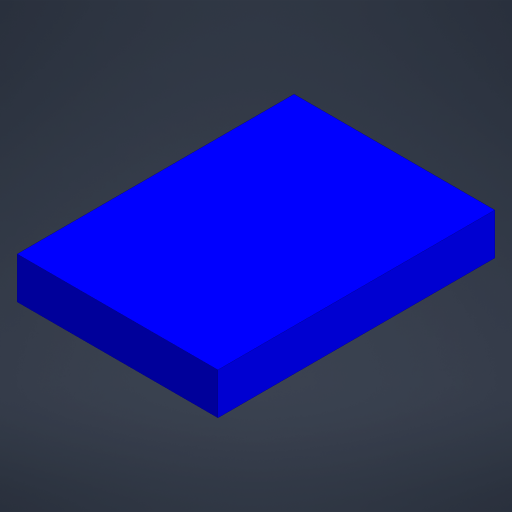
# Autodesk Inventor part: Radio
Saved by Autodesk Inventor 2024 (Build 280153000, 153)
## iProperties
Created: 2023-09-15
Part Number: Radio
Material: Radio
Document SubType Name: Modeling
Designer: Maciej
Density: 1.38 g/cm^3
Appearance: Generic
Mass: 1.2006 g
Surface Area: 7.87 cm^2
Volume: 0.87 cm^3
Author: Maciej
Autodesk Inventor part; units mm, degrees
ref_plane "YZ Plane" through (0, 0, 0) normal (1, 0, 0) x (0, 1, 0)
ref_plane "XZ Plane" through (0, 0, 0) normal (0, 1, 0) x (-1, 0, 0)
ref_plane "XY Plane" through (0, 0, 0) normal (0, 0, 1) x (1, 0, 0)
sketch "Sketch1" plane through (0, 0, 0) normal (0, 1, 0) x (-1, 0, 0)
  line L0 (-7.25, 10) -> (7.25, 10)
  line L1 (7.25, 10) -> (7.25, -10)
  line L2 (7.25, -10) -> (-7.25, -10)
  line L3 (-7.25, -10) -> (-7.25, 10)
  line L4 (-7.25, 10) -> (7.25, -10) construction
  line L5 (7.25, 10) -> (-7.25, -10) construction
  point P0 (0, 0)
  dimension "d0" = 14.5
  dimension "d1" = 20
  constraints: 12 end point, 2 midpoint, 2 parallel, 1 horizontal, 1 perpendicular
  measures "d0" distance of L1.end L2.end
  measures "d1" distance of L0.end L1.end
extrude "Extrusion1" add sketch "Sketch1" along normal blind 3
body "Solid1"
